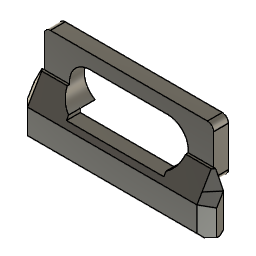
PS VITA CAP R2v4 (Autodesk Fusion 360 design; units mm, degrees)
Autodesk Fusion 360 part; units mm, degrees
note: some values were not read from the file. Set by a fixed rule: which sketch regions a step uses.
sketch "Boceto1" plane through (0, 0, 0) normal (0, 1, 0) x (1, 0, 0)
  line L0 (-6.85, -1) -> (6.85, -1)
  line L1 (6.85, -1) -> (6.85, 3.25)
  line L2 (3.15, 3.45) -> (-3.15, 3.45)
  line L3 (-6.85, 3.25) -> (-6.85, -1)
  line L4 (-3.15, 3.45) -> (-3.15, 0.15)
  line L5 (-3.15, 0.15) -> (3.15, 0.15)
  line L6 (3.15, 0.15) -> (3.15, 3.45)
  arc A0 (-3.15, 3.45) -> (-3.15, 0.15) centre (-3.15, 1.8) ccw
  arc A1 (3.15, 0.15) -> (3.15, 3.45) centre (3.15, 1.8) ccw
  line L7 (-6.85, 3.25) -> (6.85, 3.25)
  dimension "d1" = 4.25
  dimension "d2" = 3.25
  dimension "d3" = 13.7
  dimension "d4" = 6.85
  dimension "d5" = 6.3
  dimension "d6" = 3.15
  dimension "d7" = 3.3
  dimension "d55" = 3.1
  constraint horizontal L0
  constraint vertical L1
  constraint horizontal L2
  constraint vertical L3
  constraint perpendicular L2 L4
  constraint perpendicular L4 L5
  constraint perpendicular L2 L6
  constraint tangent L2 A0
  constraint tangent L2 A1
  constraint perpendicular L1 L7
  measures "d1" distance of L0.start L3.start
  measures "d2" vertical distance of origin L3.start
  measures "d3" distance of L0.start L0.end
  measures "d4" horizontal distance of origin L0.start
  measures "d5" distance of L4.end L5.end
  measures "d6" horizontal distance of origin L4.end
  measures "d7" distance of L2.end L4.end
  measures "d55" vertical distance of L3.start L4.end
extrude "Extruir1" add sketch "Boceto1" against normal blind 1.8 contours L0 L1 L3 L5 A0 A1 L7
sketch "Boceto15" plane through (0, 0, -3.25) normal (0, 0, -1) x (1, 0, 0)
  line L0 (-6.85, 0) -> (-3.9374, 0)
  line L1 (-3.9374, 0) -> (-3.9374, 1.8)
  line L2 (-3.9374, 1.8) -> (-6.85, 1.8)
  line L3 (-6.85, 1.8) -> (-6.85, 0)
  line L4 (-6.85, 1.2) -> (-3.9374, 1.2)
  dimension "d56" = 0.6
  constraint coincident L3 L4.start
  constraint coincident L1 L4.end
  constraint perpendicular L1 L4
  measures "d56" distance of L2.end L4.start
extrude "Extruir2" add sketch "Boceto15" along normal blind 3 contours L1 L2 L3 L4
extrude "Extruir3" add 1 faces at (-3.9374, -1.4, -4.25) along direction (1, 0, 0) blind 10.787
sketch "Boceto12" plane through (0, -1.8, 0) normal (0, -1, 0) x (1, 0, 0)
  arc A0 (-3.15, -0.15) -> (-3.9374, -3.25) centre (-3.15, -1.8) ccw
  line L0 (-3.15, -0.15) -> (3.15, -0.15)
  arc A1 (3.9374, -3.25) -> (3.15, -0.15) centre (3.15, -1.8) ccw
  line L1 (-6.85, -6.25) -> (6.8496, -6.25)
  line L2 (6.8496, -6.25) -> (6.8496, -3.25)
  line L3 (3.9374, -3.25) -> (-3.9374, -3.25)
  line L4 (6.8496, -3.25) -> (6.85, -3.25)
  line L5 (6.85, -3.25) -> (6.85, 1)
  line L6 (6.85, 1) -> (-6.85, 1)
  line L7 (-6.85, 1) -> (-6.85, -6.25)
  line L8 (6.85, -2.25) -> (4.7375, -2.25)
  line L9 (-4.7375, -2.25) -> (-6.85, -2.25)
  point P0 (6.8496, -3.25)
  point P1 (6.85, -2.25)
  dimension "d57" = 3
  dimension "d58" = 1
  dimension "d59" = 3
  constraint coincident L2 P0
  constraint coincident L5 P1
  constraint coincident P1 L8.start
  constraint coincident L7 L9.end
  constraint perpendicular L7 L8
  constraint coincident A1 L8.end
  constraint coincident A0 L9.start
  constraint collinear L8 L9
  measures "d57" distance of L1.end P0
  measures "d58" vertical distance of P0 P1
  measures "d59" vertical distance of A1.start L1.end
extrude "Extruir16" add sketch "Boceto12" along normal blind 0.75 contours A0 A1 L1 L2 L3 L5 L7 L8 L9
sketch "Boceto16" plane through (-6.85, 0, 0) normal (-1, 0, 0) x (0, -1, 0)
  line L0 (1.8, -2.25) -> (1.8, 1)
  line L1 (1.8, 1) -> (0, 1)
  line L2 (0, 1) -> (0, -3.25)
  line L3 (0, -3.25) -> (1.2, -3.25)
  line L4 (1.2, -3.25) -> (1.2, -6.25)
  line L5 (1.2, -6.25) -> (2.55, -6.25)
  line L6 (2.55, -6.25) -> (2.55, -2.25)
  line L7 (1.2, 1) -> (1.2, -2)
  line L8 (1.2, -2) -> (0, -2)
  line L9 (1.2, -2) -> (1.4, -2)
  line L10 (2.55, -2.25) -> (1.8, -2.25)
  line L11 (1.4, -2) -> (2.55, -3.95)
  line L12 (1.2, -2) -> (1.2, -3.25)
  point P0 (2.55, -3.95)
  dimension "d62" = 0.6
  dimension "d63" = 3
  dimension "d64" = 0.2
  dimension "d65" = 1.7
  constraint coincident L1 L7.start
  constraint perpendicular L1 L7
  constraint coincident L2 L8.end
  constraint perpendicular L2 L8
  constraint perpendicular L7 L9
  constraint coincident L6 P0
  constraint coincident P0 L11.end
  constraint coincident L3.end L4.start
  measures "d62" distance of L0.end L7.start
  measures "d63" distance of L1.end L8.end
  measures "d64" distance of L7.end L9.end
  measures "d65" distance of L6.end P0
extrude "Extruir13" cut sketch "Boceto16" against normal blind 20 contours L0 L1 L6 L7 L9 L10 L11
extrude "Extruir14" add sketch "Boceto16" along normal blind 0.8 contours L4 L5 L6 L9 L11 L12
sketch "Boceto17" plane through (6.85, 0, 0) normal (1, 0, 0) x (0, 1, 0)
  line L0 (-1.4, -2) -> (-2.1372, -3.25)
  line L1 (-2.1372, -3.25) -> (0, -3.25)
  line L2 (0, -3.25) -> (0, 1)
  line L3 (0, 1) -> (-1.2, 1)
  line L4 (-1.2, 1) -> (-1.2, -2)
  line L5 (-1.2, -2) -> (-1.4, -2)
  line L6 (-1.2064, -3.25) -> (-1.2064, -3.2)
  line L7 (-1.2064, -3.2) -> (-1.2, -2)
  constraint coincident L1 L6.start
  constraint perpendicular L1 L6
  constraint coincident L4.end L5.start
extrude "Extruir17" add sketch "Boceto17" along normal blind 0.8 contours L0 L1 L5 L6 L7
extrude "Extruir19" add 1 faces at (6.8496, -1.6521, -4.4833) along direction (1, 0, 0) blind 0.8
fillet "Empalme3" radius 0.5 4 edges at (6.85, -0.6, -3.25) (6.85, -0.6, 1) (-6.85, -0.6, 1) (-6.85, -0.6, -3.25)
chamfer "Chaflán5" distance 0.8 angle 45 5 edges at (7.6496, -2.55, -5.1) (-7.65, -2.55, -5.1) (7.6496, -2.3436, -3.6) (7.65, -1.7686, -2.625) (-7.65, -1.975, -2.975)
chamfer "Chaflán4" distance 0.3 angle 45 2 edges at (-0.0002, -2.55, -6.25) (-0.0002, -1.2, -6.25)
extrude "Extruir20" cut 1 faces at (1.3125, -1.8248, -3.25) along direction (0, 0, -1) blind 0.3
extrude "Extruir21" cut 1 faces at (-1.3125, -2.1372, -3.45) along direction (0, -1, 0) blind 1
equation "d1 = 3.25 mm + 1 mm"
equation "d4 = d3 / 2"
equation "d5 = 9.3 mm - 3 mm"
equation "d6 = d5 / 2"
equation "d57 = d59"
